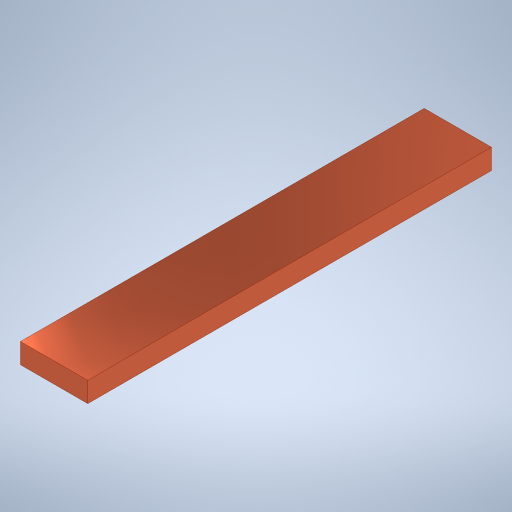
# Autodesk Inventor part: KontaktGreifer
Saved by Autodesk Inventor 2023 (Build 270158000, 158)
## iProperties
Created: 2022-12-19
Part Number: KontaktGreifer
Material: Water
Document SubType Name: Modeling
Designer: redii
Density: 0.9983 g/cm^3
Appearance: Metal 1400F Hot
Author: redii
Autodesk Inventor part; units mm, degrees
ref_plane "YZ Plane" through (0, 0, 0) normal (1, 0, 0) x (0, 1, 0)
ref_plane "XZ Plane" through (0, 0, 0) normal (0, 1, 0) x (-1, 0, 0)
ref_plane "XY Plane" through (0, 0, 0) normal (0, 0, 1) x (1, 0, 0)
sketch "Sketch1" plane through (0, 0, 0) normal (0, 1, 0) x (-1, 0, 0)
  line L0 (0, 0) -> (0.1, 0)
  line L1 (0.1, 0) -> (0.1, -0.6)
  line L2 (0.1, -0.6) -> (0, -0.6)
  line L3 (0, -0.6) -> (0, 0)
  dimension "d0" = 0.6
  dimension "d1" = 0.1
  constraints: 8 end point, 2 parallel, 1 horizontal, 1 perpendicular
  measures "d0" distance of L0.end L1.end
  measures "d1" distance of L1.end L2.end
extrude "Extrusion1" add sketch "Sketch1" along normal blind 0.03
body "Solid1"
